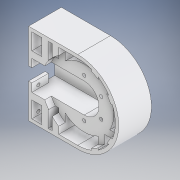
# Autodesk Inventor part: SJ001
Saved by Autodesk Inventor 2017 SP1 (Build 210196100, 196)
## iProperties
Created: 2017-06-03
Part Number: SJ001
Material: ABS Plastic
Document SubType Name: Modeling
Designer: Zach
Density: 1.06 g/cm^3
Appearance: CR White
Author: Zach
Autodesk Inventor part; units mm, degrees
ref_plane "YZ Plane" through (0, 0, 0) normal (1, 0, 0) x (0, 1, 0)
ref_plane "XZ Plane" through (0, 0, 0) normal (0, 1, 0) x (-1, 0, 0)
ref_plane "XY Plane" through (0, 0, 0) normal (0, 0, 1) x (1, 0, 0)
sketch "Sketch1" plane through (0, 0, 0) normal (0, 0, 1) x (1, 0, 0)
  circle A0 centre (0, 0) radius 62.5 construction
  line L0 (0, 62.5) -> (-75, 62.5)
  line L1 (-75, 62.5) -> (-75, -62.5)
  line L2 (-75, -62.5) -> (0, -62.5)
  arc A1 (0, -62.5) -> (0, 62.5) centre (0, 0) ccw
  dimension "d0" = 125
  dimension "d1" = 75
  constraints: 6 end point, 4 point on circle, 4 tangent, 2 centre point, 2 vertical alignment, 1 coincident, 1 concentric, 1 horizontal, 1 perpendicular
  measures "d0" diameter of A0
  measures "d1" distance of L0.start L0.end
extrude "Extrusion1" add sketch "Sketch1" along normal blind 50
sketch "Sketch6" plane through (0, 0, 50) normal (0, 0, 1) x (1, 0, 0)
  circle A0 centre (0, 0) radius 22.5
  arc A1 (0, -62.5) -> (0, 62.5) centre (0, 0) ccw projected
  dimension "d125" = 45
  constraints: 1 centre point, 1 coincident
  measures "d125" diameter of A0
extrude "Extrusion6" cut sketch "Sketch6" against normal blind 40
sketch "Sketch7" plane through (0, 0, 50) normal (0, 0, 1) x (1, 0, 0)
  line L0 (0, 10) -> (-75, 10)
  line L1 (-75, 10) -> (-75, -10)
  line L2 (-75, -10) -> (0, -10)
  line L3 (0, -10) -> (0, 10)
  circle A0 centre (0, 0) radius 22.5 projected
  line L4 (-75, 62.5) -> (-75, -62.5) projected
  point P0 (-75, 0)
  dimension "d28" = 20
  constraints: 8 end point, 3 midpoint, 2 parallel, 1 coincident, 1 horizontal, 1 perpendicular
  measures "d28" distance of L1.end L0.end
extrude "Extrusion7" cut sketch "Sketch7" against normal blind 40 contours L3 L2 A0 L0 | A0 L2 L1 L0 picked at (-7.5, 0)
sketch "Sketch9" plane through (0, 0, 50) normal (0, 0, 1) x (1, 0, 0)
  circle A0 centre (0, 30) radius 2.5
  circle A1 centre (-25.9808, 15) radius 2.5
  circle A2 centre (-25.9808, -15) radius 2.5
  circle A3 centre (0, -30) radius 2.5
  circle A4 centre (25.9808, -15) radius 2.5
  circle A5 centre (25.9808, 15) radius 2.5
  circle A6 centre (0, 0) radius 30 construction
  dimension "d123" = 60
  dimension "d35" = 5
  dimension "d39" = 360
  constraints: 6 centre point, 2 vertical alignment, 1 coincident, 15 other
  measures "d35" diameter of A0
extrude "Extrusion9" cut sketch "Sketch9" against normal through all
sketch "Sketch10" plane through (0, 0, 50) normal (0, 0, 1) x (1, 0, 0)
  circle A0 centre (0, 0) radius 45
  arc A1 (0, -57.5) -> (0, -57.5) centre (0, 0) ccw
  line L0 (0, -57.5) -> (-70, -57.5)
  line L1 (-70, 57.5) -> (-70, -57.5)
  line L2 (0, -57.5) -> (-75, -57.5)
  line L3 (0, 57.5) -> (-70, 57.5)
  circle A2 centre (0, 0) radius 57.5 construction
  arc A3 (0, -57.5) -> (0, 57.5) centre (0, 0) ccw
  line L4 (0, 62.5) -> (-75, 62.5) construction
  line L5 (-75, 62.5) -> (-75, 10) construction
  line L6 (-75, -10) -> (-75, 10) construction
  line L7 (-75, -10) -> (-75, -62.5) construction
  line L8 (-75, -62.5) -> (0, -62.5) construction
  arc A4 (0, -62.5) -> (0, 62.5) centre (0, 0) ccw construction
  point P0 (-70, 0)
  dimension "d111" = 115
  dimension "d43" = 90
  dimension "d114" = 90
  dimension "d124" = 5
  dimension "d212" = 5
  dimension "d213" = 5
  constraints: 8 end point, 4 point on circle, 3 centre point, 3 coincident, 2 tangent, 1 midpoint, 1 perpendicular, 1 vertical alignment, 3 other
  measures "d43" diameter of A0
  measures "d114" angle of L1 L3
  measures "d124" distance between parallel lines of L4 L3
  measures "d212" distance between parallel lines of L8 L0
  measures "d213" distance from line of L6 point (-70, 0)
extrude "Extrusion10" cut sketch "Sketch10" against normal blind 40
sketch "Sketch18" plane through (-75, -62.5, 0) normal (-1, 0, 0) x (0, 0, 1)
  circle A0 centre (40, 45) radius 2.5
  circle A1 centre (20, 45) radius 2.5
  line L0 (0, 125) -> (0, 0)
  circle A2 centre (40, 80) radius 2.5
  circle A3 centre (20, 80) radius 2.5
  circle A4 centre (20, 115) radius 2.5
  circle A5 centre (20, 10) radius 2.5
  circle A6 centre (40, 10) radius 2.5
  circle A7 centre (40, 115) radius 2.5
  line L1 (0, 125) -> (50, 125)
  line L2 (0, 0) -> (50, 0)
  line L3 (40, 10) -> (20, 10) construction
  line L4 (40, 115) -> (20, 115) construction
  line L5 (40, 45) -> (20, 45) construction
  line L6 (40, 80) -> (20, 80) construction
  line L7 (50, 52.5) -> (10, 52.5) projected
  line L8 (10, 72.5) -> (50, 72.5) projected
  point P0 (0, 62.5)
  point P1 (30, 115)
  point P2 (30, 80)
  point P3 (30, 45)
  point P4 (30, 10)
  point P5 (30, 52.5)
  dimension "d76" = 5
  dimension "d77" = 5
  dimension "d80" = 20
  dimension "d91" = 5
  dimension "d92" = 5
  dimension "d94" = 5
  dimension "d95" = 5
  dimension "d96" = 5
  dimension "d97" = 5
  dimension "d115" = 10
  dimension "d118" = 10
  dimension "d271" = 7.5
  dimension "d272" = 7.5
  constraints: 14 end point, 10 vertical alignment, 8 centre point, 5 midpoint, 4 coincident, 4 horizontal alignment, 3 horizontal
  measures "d76" diameter of A0
  measures "d77" diameter of A1
  measures "d80" distance of L5.end L5.start
  measures "d91" diameter of A2
  measures "d92" diameter of A3
  measures "d94" diameter of A4
  measures "d95" diameter of A5
  measures "d96" diameter of A6
  measures "d97" diameter of A7
  measures "d115" distance from line of L1 L4.start
  measures "d118" distance from line of L2 L3.start
  measures "d271" distance between parallel lines of L7 L5
  measures "d272" distance between parallel lines of L6 L8
extrude "Extrusion39" cut sketch "Sketch18" against normal blind 10
sketch "Sketch46" plane through (0, 0, 10) normal (0, 0, 1) x (1, 0, 0)
  arc A0 (-43.8748, -10) -> (-43.8748, 10) centre (0, 0) ccw construction
  line L0 (-45, 22.5) -> (-70, 22.5)
  line L1 (-31.1247, 32.5) -> (-70, 32.5)
  line L2 (-70, 32.5) -> (-70, 22.5)
  line L3 (-70, 22.5) -> (-31.1247, 22.5)
  line L4 (-31.1247, 22.5) -> (-31.1247, 32.5)
  line L5 (-120.4871, 0) -> (150.4871, 0) construction
  line L6 (-95, 57.5) -> (0, 57.5) construction
  line L7 (-38.9711, 22.5) -> (-28.9711, 22.5)
  line L8 (-28.9711, 22.5) -> (-28.9711, 57.5)
  line L9 (-28.9711, 57.5) -> (-38.9711, 57.5)
  line L10 (-38.9711, 57.5) -> (-38.9711, 22.5)
  arc A1 (0, -57.5) -> (0, 57.5) centre (0, 0) ccw construction
  line L11 (31.1247, 32.5) -> (52.915, 32.5)
  line L12 (52.915, 32.5) -> (52.915, 22.5)
  line L13 (52.915, 22.5) -> (31.1247, 22.5)
  line L14 (31.1247, 22.5) -> (31.1247, 32.5)
  line L15 (31.1247, 22.5) -> (21.1247, 22.5)
  line L16 (21.1247, 22.5) -> (21.1247, 53.4789)
  line L17 (21.1247, 53.4789) -> (31.1247, 53.4789)
  line L18 (31.1247, 53.4789) -> (31.1247, 22.5)
  line L19 (-45, -22.5) -> (-70, -22.5)
  line L20 (-31.1247, -32.5) -> (-70, -32.5)
  line L21 (-70, -32.5) -> (-70, -22.5)
  line L22 (-70, -22.5) -> (-31.1247, -22.5)
  line L23 (-31.1247, -22.5) -> (-31.1247, -32.5)
  line L24 (-28.9711, -22.5) -> (-28.9711, -57.5)
  line L25 (-28.9711, -57.5) -> (-38.9711, -57.5)
  line L26 (-38.9711, -57.5) -> (-38.9711, -22.5)
  line L27 (31.1247, -32.5) -> (52.915, -32.5)
  line L28 (52.915, -32.5) -> (52.915, -22.5)
  line L29 (52.915, -22.5) -> (31.1247, -22.5)
  line L30 (31.1247, -22.5) -> (31.1247, -32.5)
  line L31 (31.1247, -22.5) -> (21.1247, -22.5)
  line L32 (21.1247, -22.5) -> (21.1247, -53.4789)
  line L33 (21.1247, -53.4789) -> (31.1247, -53.4789)
  line L34 (31.1247, -53.4789) -> (31.1247, -22.5)
  line L35 (-28.9711, -22.5) -> (-38.9711, -22.5)
  line L36 (-70, -22.5) -> (27.5, -22.5) construction
  line L37 (-70, 10) -> (-70, 57.5) construction
  arc A2 (-43.8748, -10) -> (-43.8748, 10) centre (0, 0) ccw projected
  line L38 (-50.5624, 22.5) -> (-50.5624, -22.5) construction
  point P0 (15, 0)
  point P1 (15, 0)
  point P2 (31.1247, 37.9895)
  point P3 (31.1247, -37.9895)
  point P4 (21.1247, 37.9895)
  point P5 (21.1247, -37.9895)
  point P6 (-50.5624, 0)
  dimension "d229" = 10
  dimension "d230" = 10
  dimension "d231" = 10
  dimension "d232" = 10
  constraints: 76 end point, 15 symmetric about line, 11 point on circle, 8 parallel, 7 midpoint, 5 horizontal, 5 perpendicular, 5 point on line, 2 centre point, 2 vertical alignment, 1 coincident, 1 collinear, 1 horizontal alignment
  measures "d229" distance of L1.end L0.end
  measures "d230" distance of L9.end L8.end
  measures "d231" distance of L11.end L12.end
  measures "d232" distance of L16.end L17.end
extrude "Extrusion44" add sketch "Sketch46" along normal blind 40
sketch "Sketch22" plane through (0, 0, 50) normal (0, 0, 1) x (1, 0, 0)
  arc A0 (0, -62.5) -> (0, 62.5) centre (0, 0) ccw projected
  circle A1 centre (0, 0) radius 55
  point P0 (0, 0)
  dimension "d122" = 110
  constraints: 1 centre point, 1 coincident
  measures "d122" diameter of A1
extrude "Extrusion20" cut sketch "Sketch22" against normal blind 10
sketch "Sketch53" plane through (0, 0, 10) normal (0, 0, 1) x (1, 0, 0)
  line L0 (-70, 57.5) -> (-38.9711, 57.5) projected
  line L1 (-70, 32.5) -> (-38.9711, 32.5) projected
  line L2 (-55, 57.5) -> (-45, 57.5)
  line L3 (-45, 57.5) -> (-45, 32.5)
  line L4 (-45, 32.5) -> (-55, 32.5)
  line L5 (-55, 32.5) -> (-55, 57.5)
  line L6 (-70, 32.5) -> (-70, 57.5) projected
  line L7 (-70, -32.5) -> (-44.3706, -32.5) projected
  line L8 (-38.9711, -57.5) -> (-70, -57.5) projected
  line L9 (-55, -32.5) -> (-45, -32.5)
  line L10 (-45, -32.5) -> (-45, -57.5)
  line L11 (-45, -57.5) -> (-55, -57.5)
  line L12 (-55, -57.5) -> (-55, -32.5)
  point P0 (0, 0)
  point P1 (-45, -45)
  point P2 (-45, 45)
  point P3 (-55, -45)
  point P4 (-55, 45)
  dimension "d254" = 10
  dimension "d255" = 15
  constraints: 16 end point, 4 midpoint, 4 parallel, 4 point on line, 2 horizontal, 2 perpendicular, 2 vertical alignment
  measures "d254" distance between parallel lines of L5 L3
  measures "d255" distance between parallel lines of L6 L5
extrude "Extrusion50" add sketch "Sketch53" along normal blind 40 contours L0 L3 L1 L5 | L7 L10 L8 L12
sketch "Sketch54" plane through (-75, 62.5, 0) normal (-1, 0, 0) x (0, 0, 1)
  circle A0 centre (40, -10) radius 2.5 projected
  circle A1 centre (20, -10) radius 2.5 projected
  circle A2 centre (40, -45) radius 2.5 projected
  circle A3 centre (20, -45) radius 2.5 projected
  circle A4 centre (40, -80) radius 2.5 projected
  circle A5 centre (20, -80) radius 2.5 projected
  circle A6 centre (20, -115) radius 2.5 projected
  circle A7 centre (40, -115) radius 2.5 projected
  point P0 (0, -62.5)
extrude "Extrusion51" cut sketch "Sketch54" against normal blind 30
sketch "Sketch57" plane through (0, 0, 40) normal (0, 0, 1) x (1, 0, 0)
  arc A0 (-38.9711, 22.5) -> (-43.8748, 10) centre (0, 0) ccw construction
  line L0 (-38.9711, 22.5) -> (0, 22.5)
  arc A1 (-20.1556, -10) -> (-20.1556, 10) centre (0, 0) ccw construction
  line L1 (-50.1871, -22.5) -> (-38.9711, -22.5) construction
  line L2 (-38.9711, -22.5) -> (0, -22.5)
  arc A2 (0, -22.5) -> (0, 22.5) centre (0, 0) ccw
  arc A3 (-38.9711, 22.5) -> (-43.8748, 10) centre (0, 0) ccw projected
  arc A4 (-43.8748, -10) -> (-38.9711, -22.5) centre (0, 0) ccw projected
  arc A5 (-38.9711, 22.5) -> (-38.9711, -22.5) centre (0, 0) ccw
  constraints: 6 point on circle, 4 end point, 3 tangent, 2 centre point, 1 horizontal
extrude "Extrusion54" cut sketch "Sketch57" against normal blind 30
sketch "Sketch58" plane through (0, 0, 0) normal (0, 0, -1) x (-1, 0, 0)
  circle A0 centre (0, 30) radius 2.5 projected
  circle A1 centre (25.9808, 15) radius 2.5 projected
  circle A2 centre (25.9808, -15) radius 2.5 projected
  circle A3 centre (0, -30) radius 2.5 projected
  circle A4 centre (-25.9808, -15) radius 2.5 projected
  circle A5 centre (-25.9808, 15) radius 2.5 projected
  point P0 (0, 0)
extrude "Extrusion55" add sketch "Sketch58" against normal blind 10
sketch "Sketch60" plane through (-75, -62.5, 0) normal (-1, 0, 0) x (0, 0, 1)
  line L0 (24.8425, 40) -> (10, 40)
  line L1 (10, 40) -> (10, 85)
  line L2 (10, 85) -> (24.8425, 85)
  line L3 (24.8425, 85) -> (24.8425, 40)
  line L4 (10, 52.5) -> (10, 72.5) projected
  line L5 (40, 85) -> (50, 85) projected
  line L6 (10, 85) -> (50, 85) projected
  line L7 (10, 85) -> (40, 85) projected
  line L8 (10, 40) -> (40, 40) projected
  line L9 (50, 40) -> (10, 40) projected
  line L10 (50, 40) -> (40, 40) projected
  point P0 (0, 62.5)
  point P1 (50, 62.5)
  point P2 (10, 62.5)
  dimension "d273" = 14.8425
  constraints: 8 end point, 2 midpoint, 2 parallel, 1 horizontal, 1 horizontal alignment, 1 perpendicular, 1 point on line
  measures "d273" distance of L0.start L0.end
extrude "Extrusion56" cut sketch "Sketch60" against normal blind 5
sketch "Sketch61" plane through (0, 0, 10) normal (0, 0, 1) x (1, 0, 0)
  circle A0 centre (0, 0) radius 4
  circle A1 centre (-40.5, 0) radius 4
  dimension "d277" = 8
  dimension "d278" = 8
  dimension "d279" = 40.5
  constraints: 2 centre point, 1 coincident, 1 horizontal alignment
  measures "d277" diameter of A0
  measures "d278" diameter of A1
  measures "d279" distance of point (0, 0) A1.centre
extrude "Extrusion57" cut sketch "Sketch61" against normal through all
body "Solid1"
